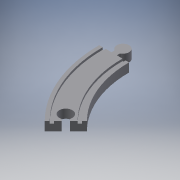
# Autodesk Inventor part: CurvedTrack
Saved by Autodesk Inventor 2016 (Build 200138000, 138)
## iProperties
Created: 2012-11-27
Part Number: CurvedTrack
Material: Generic
Document SubType Name: Modeling
Designer: choueugene
Density: 1 g/cm^3
Appearance: Default
Author: choueugene
Autodesk Inventor part; units mm, degrees
ref_plane "YZ Plane" through (0, 0, 0) normal (1, 0, 0) x (0, 1, 0)
ref_plane "XZ Plane" through (0, 0, 0) normal (0, 1, 0) x (-1, 0, 0)
ref_plane "XY Plane" through (0, 0, 0) normal (0, 0, 1) x (1, 0, 0)
sketch "MainSketch1" plane through (0, 0, 0) normal (0, 0, 1) x (1, 0, 0)
  line L0 (0, 0) -> (86.36, 0)
  line L1 (86.36, 0) -> (86.36, 25.4)
  line L2 (86.36, 25.4) -> (76.2, 25.4)
  line L3 (76.2, 25.4) -> (76.2, 19.05)
  line L4 (76.2, 19.05) -> (67.31, 19.05)
  line L5 (67.31, 19.05) -> (67.31, 25.4)
  line L6 (67.31, 25.4) -> (19.05, 25.4)
  line L7 (19.05, 25.4) -> (19.05, 19.05)
  line L8 (19.05, 19.05) -> (10.16, 19.05)
  line L9 (10.16, 19.05) -> (10.16, 25.4)
  line L10 (10.16, 25.4) -> (0, 25.4)
  line L11 (0, 25.4) -> (0, 0)
  line L12 (381, 0) -> (381, 63.5) construction
  dimension "d0" = 86.36
  dimension "d1" = 10.16
  dimension "d2" = 19.05
  dimension "d3" = 67.31
  dimension "d4" = 76.2
  dimension "d5" = 19.05
  dimension "d6" = 25.4
  dimension "d7" = 25.4
  dimension "d8" = 19.05
  dimension "d9" = 25.4
  dimension "d10" = 381
  dimension "d30" = 63.5
  constraints: 26 end point, 11 parallel, 1 horizontal, 1 horizontal alignment, 1 perpendicular
  measures "d0" distance of L0.start L0.end
  measures "d1" distance of L9.end L10.end
  measures "d2" horizontal distance of L0.start L7.end
  measures "d3" horizontal distance of L0.start L5.end
  measures "d4" horizontal distance of L0.start L2.end
  measures "d5" vertical distance of L0.start L8.end
  measures "d6" distance of L10.end L0.start
  measures "d7" vertical distance of L0.start L6.end
  measures "d8" vertical distance of L0.start L3.end
  measures "d9" distance of L0.end L1.end
  measures "d10" distance from line of L12 L0.start
  measures "d30" distance of L12.start L12.end
revolve "MainRevolution1" add sketch "MainSketch1" angle 45 about axis through (381, 0, 0) along (0, 1, 0)
sketch "HeadSketch" plane through (19.05, 25.4, 0) normal (0, 1, 0) x (1, 0, 0)
  line L0 (48.26, 0) -> (0, 0) projected
  arc A0 (31.75, 9.3356) -> (16.51, 9.3356) centre (24.13, 25.4) ccw
  arc A1 (-19.05, 0) -> (92.5423, -269.4077) centre (361.95, 0) ccw projected
  arc A2 (67.31, 0) -> (153.6081, -208.3419) centre (361.95, 0) ccw projected
  line L1 (-8.89, 0) -> (-19.05, 0) projected
  line L2 (67.31, 0) -> (57.15, 0) projected
  line L3 (57.15, 0) -> (48.26, 0) projected
  line L4 (0, 0) -> (-8.89, 0) projected
  line L5 (92.5423, -269.4077) -> (99.7265, -262.2235) projected
  line L6 (99.7265, -262.2235) -> (106.0127, -255.9373) projected
  line L7 (140.1377, -221.8123) -> (146.4239, -215.5261) projected
  line L8 (146.4239, -215.5261) -> (153.6081, -208.3419)
  line L9 (16.51, 0) -> (31.75, 0)
  line L10 (31.75, 0) -> (31.75, 9.3356)
  line L11 (16.51, 9.3356) -> (16.51, 0)
  line L12 (106.0127, -255.9373) -> (140.1377, -221.8123) projected
  arc A3 (123.0945, -227.2198) -> (111.4202, -238.8941) centre (105.1174, -220.917) ccw
  line L13 (128.9124, -233.0376) -> (123.0945, -227.2198)
  line L14 (111.4202, -238.8941) -> (117.238, -244.712)
  line L15 (117.238, -244.712) -> (128.9124, -233.0376)
  line L16 (123.0945, -227.2198) -> (111.4202, -238.8941) construction
  line L17 (105.1174, -220.917) -> (123.0752, -238.8748) construction
  point P0 (24.13, 0)
  dimension "d12" = 43.18
  dimension "d13" = 25.4
  dimension "d14" = 35.56
  dimension "d15" = 15.24
  dimension "d16" = 43.18
  dimension "d26" = 38.1
  dimension "d27" = 16.51
  dimension "d32" = 90
  dimension "d33" = 90
  dimension "d34" = 17.9578
  constraints: 18 end point, 4 point on circle, 4 point on line, 3 midpoint, 3 perpendicular, 2 centre point, 2 parallel, 1 horizontal
  measures "d12" horizontal distance of A0.centre L1.end
  measures "d13" distance from line of A0.centre L0
  measures "d14" diameter of A0
  measures "d15" distance of L9.start L9.end
  measures "d16" distance of point (24.13, 0) L1.end
  measures "d26" diameter of A3
  measures "d27" distance of L14.end L13.start
  measures "d32" angle of L13 L12
  measures "d33" angle of L16 L13
  measures "d34" horizontal distance of L17.start L17.end
extrude "TopHeadExtrusion1" add sketch "HeadSketch" against normal blind 25.4 contours L0 L11 A0 L10
extrude "BottomHeadCut" cut sketch "HeadSketch" against normal through all contours L12 L14 A3 L13
fillet "NeckFillet" radius 4.826 4 edges at (50.8, 12.7, -9.3356) (35.56, 12.7, -9.3356) (142.1445, 12.7, 227.2198) (130.4702, 12.7, 238.8941)
body "Solid1"
